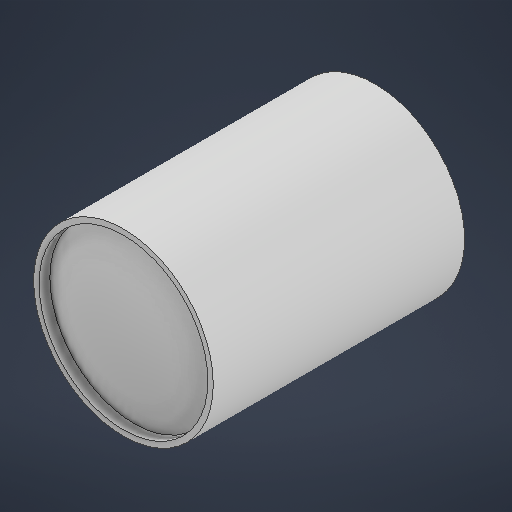
# Autodesk Inventor part: 35mmLens
Saved by Autodesk Inventor 2026.2 (Build 302298000, 298)
## iProperties
Created: 2026-02-27
Part Number: 35mmLens
Material: Generic
Document SubType Name: Modeling
Designer: mumin
Density: 1 g/cm^3
Appearance: Default
Author: mumin
Autodesk Inventor part; units mm, degrees
ref_plane "YZ Plane" through (0, 0, 0) normal (1, 0, 0) x (0, 1, 0)
ref_plane "XZ Plane" through (0, 0, 0) normal (0, 1, 0) x (-1, 0, 0)
ref_plane "XY Plane" through (0, 0, 0) normal (0, 0, 1) x (1, 0, 0)
sketch "Sketch1" plane through (0, 0, 0) normal (0, 0, 1) x (1, 0, 0)
  circle A0 centre (0, 0) radius 25
  dimension "d0" = 50
  constraints: 1 centre point, 1 coincident
  measures "d0" diameter of A0
extrude "Lens Body" add sketch "Sketch1" along normal blind 70
sketch "Sketch2" plane through (0, 0, 0) normal (0, 0, -1) x (-1, 0, 0)
  circle A0 centre (0, 0) radius 12.45
  circle A1 centre (0, 0) radius 10.95
  dimension "d3" = 24.9
  dimension "d4" = 1.5
  constraints: 2 centre point, 1 coincident
  measures "d3" diameter of A0
  measures "d4" radial gap between concentric circles of A0 A1
extrude "Camera Mount" add sketch "Sketch2" along normal blind 5
sketch "Sketch4" plane through (0, 0, 0) normal (1, 0, 0) x (0, 1, 0)
  line L0 (25, 70) -> (-25, 70) projected
  line L1 (25, 0) -> (-25, 0) projected
  line L2 (25, 70) -> (-25, 70) projected
  line L3 (-25, 0) -> (-25, 70) projected
  line L4 (25, 70) -> (-25, 70)
  line L5 (-25, 70) -> (-25, 67)
  line L6 (-25, 67) -> (25, 67)
  line L7 (25, 67) -> (25, 70)
  line L8 (25, 70) -> (-25, 70) projected
  line L9 (23.5, 70) -> (23.5, 67)
  line L10 (0, 70) -> (0, 67)
  line L11 (-23.5, 70) -> (-23.5, 67)
  arc A0 (23.5, 67) -> (-23.5, 67) centre (0, 3.1082) ccw
  line L12 (0, -20.2369) -> (0, 86.4217) projected
  point P0 (0, 0)
  point P1 (12.6451, 70)
  point P2 (0, 71.1847)
  dimension "d7" = 3
  dimension "d8" = 47
  constraints: 14 end point, 3 point on line, 2 midpoint, 2 parallel, 2 perpendicular, 2 point on circle, 2 symmetric about line, 1 centre point, 1 horizontal
  measures "d7" distance of L5.end L4.end
  measures "d8" diameter of L9 L10
revolve "Remove Material" cut sketch "Sketch4" angle 360 about axis through (0, 0, -10) along (0, 0, 1) contours L9 A0 L0
revolve "Convex Lens Shape" add sketch "Sketch4" angle 360 about axis through (0, 0, -10) along (0, 0, 1) picked at (7.0342, 70.2191) contours L0 L12 A0
body "Solid1"
